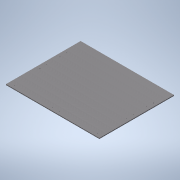
# Autodesk Inventor part: Base
Saved by Autodesk Inventor 2022 (Build 260153000, 153)
## iProperties
Created: 2021-09-08
Part Number: Base
Material: Steel, Mild, Welded
Document SubType Name: Modeling
Designer: Andres
Density: 7.85 g/cm^3
Appearance: Weld - Steel Mild
Author: Andres
Autodesk Inventor part; units mm, degrees
ref_plane "YZ Plane" through (0, 0, 0) normal (1, 0, 0) x (0, 1, 0)
ref_plane "XZ Plane" through (0, 0, 0) normal (0, 1, 0) x (-1, 0, 0)
ref_plane "XY Plane" through (0, 0, 0) normal (0, 0, 1) x (1, 0, 0)
sketch "Sketch1" plane through (0, 0, 0) normal (0, 1, 0) x (-1, 0, 0)
  line L0 (-280, -223.75) -> (280, -223.75)
  line L1 (280, -223.75) -> (280, 223.75)
  line L2 (280, 223.75) -> (-280, 223.75)
  line L3 (-280, 223.75) -> (-280, -223.75)
  line L4 (-280, -223.75) -> (280, 223.75) construction
  line L5 (280, -223.75) -> (-280, 223.75) construction
  line L6 (-280, 228.75) -> (280, 228.75)
  arc A0 (285, 223.75) -> (280, 228.75) centre (280, 223.75) ccw
  line L7 (285, 223.75) -> (285, -223.75)
  arc A1 (280, -228.75) -> (285, -223.75) centre (280, -223.75) ccw
  line L8 (280, -228.75) -> (-280, -228.75)
  arc A2 (-285, -223.75) -> (-280, -228.75) centre (-280, -223.75) ccw
  line L9 (-285, -223.75) -> (-285, 223.75)
  arc A3 (-280, 228.75) -> (-285, 223.75) centre (-280, 223.75) ccw
  point P0 (0, 0)
  point P1 (0, 0)
  dimension "d2" = 0
  dimension "d3" = 0
  dimension "d0" = 560
  dimension "d1" = 447.5
  dimension "espesor" = 5
  constraints: 20 end point, 8 point on circle, 8 point on line, 5 horizontal, 4 centre point, 4 midpoint, 4 parallel, 4 vertical, 2 perpendicular, 23 other
  measures "d0" distance of L4.end L5.end
  measures "d1" distance between parallel lines of L0 L2
  measures "espesor" distance between parallel lines of L1 L7
extrude "Extrusion1" add sketch "Sketch1" along normal blind 5 contours L3 L2 L1 L0
sketch "Sketch2" plane through (0, 5, 0) normal (0, 1, 0) x (1, 0, 0)
  line L0 (-290, -203.75) -> (-250, -203.75) construction
  line L1 (-280, -223.75) -> (280, -223.75) construction
  line L2 (0, 313.25) -> (0, -313.25) construction
  line L3 (290, -203.75) -> (250, -203.75) construction
  line L4 (-260, 120) -> (-260, 80) construction
  line L5 (-260, 0) -> (-260, -40) construction
  line L6 (-280, 223.75) -> (-280, -223.75) construction
  line L7 (260, 120) -> (260, 80) construction
  line L8 (260, 0) -> (260, -40) construction
  point P0 (0, 0)
  point P1 (-300, -150)
  point P2 (280, -223.75)
  point P3 (-20, -203.75)
  point P4 (20, -203.75)
  dimension "d7" = 40
  dimension "d8" = 20
  dimension "d9" = 500
  dimension "d10" = 40
  dimension "d11" = 40
  dimension "d12" = 80
  dimension "d14" = 20
  dimension "d23" = 40
  constraints: 12 end point, 7 symmetric about line, 2 horizontal alignment, 2 vertical, 1 collinear, 1 horizontal, 1 other
  measures "d7" distance of L0.start L0.end
  measures "d9" distance of L3.end L0.end
  measures "d10" distance of L5.start L5.end
  measures "d11" distance of L4.start L4.end
  measures "d12" distance of L5.start L4.end
  measures "d14" distance from line of L6 L5.end
  measures "d23" distance of point (20, -203.75) point (-20, -203.75)
hole "Hole1" at (-290, 5, 203.75) at (-250, 5, 203.75) at (290, 5, 203.75) at (250, 5, 203.75) at (-260, 5, -120) at (-260, 5, -80) at (-260, 5, 40) at (-260, 5, 0) at (260, 5, -120) at (260, 5, -80) at (260, 5, 0) at (260, 5, 40) at (-20, 5, 203.75) at (20, 5, 203.75) direction (0, -1, 0) diameter 3.4 end through all clearance for "Socket Head Cap Screw ISO 4762" size "M3" standard "ISO"
equation "\"d4\" = espesor"
equation "\"d10\" = d7"
equation "\"d11\" = d7"
equation "\"d23\" = d7"
body "Solid1"
